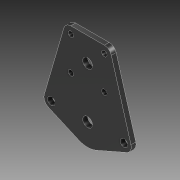
# Autodesk Inventor part: Dog Shifter Reverse Plate
Saved by Autodesk Inventor 2021 (Build 250183000, 183)
## iProperties
Created: 2021-04-11
Part Number: Dog Shifter Reverse Plate
Material: Aluminum 6061
Document SubType Name: Modeling
Designer: Cal
Density: 2.7 g/cm^3
Appearance: Glossy - Black
Author: Cal
Autodesk Inventor part; units mm, degrees
ref_plane "YZ Plane" through (0, 0, 0) normal (1, 0, 0) x (0, 1, 0)
ref_plane "XZ Plane" through (0, 0, 0) normal (0, 1, 0) x (-1, 0, 0)
ref_plane "XY Plane" through (0, 0, 0) normal (0, 0, 1) x (1, 0, 0)
sketch "Sketch1" plane through (0, 0, 0) normal (0, 0, 1) x (1, 0, 0)
  circle A0 centre (0, 0) radius 3.175
  circle A1 centre (23.8125, 0) radius 2.4892
  circle A2 centre (-23.8125, 0) radius 2.4892
  line L0 (-10.9601, 22.3774) -> (10.9601, 22.3774) construction
  line L1 (10.9601, 22.3774) -> (10.9601, 44.2976) construction
  line L2 (10.9601, 44.2976) -> (-10.9601, 44.2976) construction
  line L3 (-10.9601, 44.2976) -> (-10.9601, 22.3774) construction
  line L4 (-10.9601, 22.3774) -> (10.9601, 44.2976) construction
  line L5 (10.9601, 22.3774) -> (-10.9601, 44.2976) construction
  circle A3 centre (0, 33.3375) radius 3.175
  circle A4 centre (-10.9601, 44.2976) radius 1.778
  circle A5 centre (-10.9601, 22.3774) radius 1.778
  circle A6 centre (10.9601, 22.3774) radius 1.778
  circle A7 centre (10.9601, 44.2976) radius 1.778
  arc A8 (-5.715, -13.0947) -> (5.715, -13.0947) centre (0, 0) ccw
  arc A9 (-10.9601, 49.0601) -> (-15.534, 45.6247) centre (-10.9601, 44.2976) ccw
  arc A10 (15.534, 45.6247) -> (10.9601, 49.0601) centre (10.9601, 44.2976) ccw
  arc A11 (-28.3864, 1.3271) -> (-25.7175, -4.3649) centre (-23.8125, 0) ccw
  arc A12 (25.7175, -4.3649) -> (28.3864, 1.3271) centre (23.8125, 0) ccw
  line L6 (-28.3864, 1.3271) -> (-15.534, 45.6247)
  line L7 (-10.9601, 49.0601) -> (10.9601, 49.0601)
  line L8 (15.534, 45.6247) -> (28.3864, 1.3271)
  line L9 (5.715, -13.0947) -> (25.7175, -4.3649)
  line L10 (-5.715, -13.0947) -> (-25.7175, -4.3649)
  point P0 (0, 33.3375)
  dimension "d0" = 6.35
  dimension "d1" = 4.9784
  dimension "d4" = 360
  dimension "d6" = 47.625
  dimension "d7" = 21.9202
  dimension "d8" = 6.35
  dimension "d9" = 3.556
  dimension "d12" = 360
  dimension "d14" = 33.3375
  dimension "d16" = 28.575
  dimension "d18" = 9.525
  dimension "d19" = 9.525
  constraints: 22 end point, 13 centre point, 10 point on circle, 10 tangent, 6 coincident, 3 midpoint, 2 equal radius, 2 parallel, 2 perpendicular, 1 horizontal, 1 horizontal alignment, 1 vertical alignment, 14 other
  measures "d0" diameter of A0
  measures "d1" diameter of A1
  measures "d6" distance of A1.centre A2.centre
  measures "d7" distance of L2.end L1.end
  measures "d8" diameter of A3
  measures "d9" diameter of A4
  measures "d14" distance of A3.centre A0.centre
  measures "d16" diameter of A8
  measures "d18" diameter of A11
  measures "d19" diameter of A12
extrude "Extrusion1" add sketch "Sketch1" along normal blind 3.175
body "Solid1"
